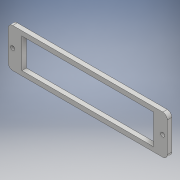
# Autodesk Inventor part: Frame
Saved by Autodesk Inventor 2017 (Build 210142000, 142)
## iProperties
Created: 2016-12-07
Part Number: Frame
Material: Generic
Document SubType Name: Modeling
Designer: willt
Density: 1 g/cm^3
Appearance: Default
Author: willt
Autodesk Inventor part; units mm, degrees
ref_plane "YZ Plane" through (0, 0, 0) normal (1, 0, 0) x (0, 1, 0)
ref_plane "XZ Plane" through (0, 0, 0) normal (0, 1, 0) x (-1, 0, 0)
ref_plane "XY Plane" through (0, 0, 0) normal (0, 0, 1) x (1, 0, 0)
sketch "Sketch2" plane through (0, 0, 0) normal (0, 1, 0) x (-1, 0, 0)
  line L0 (72.5, 16.5) -> (-72.5, 16.5)
  line L1 (-72.5, 16.5) -> (-72.5, -16.5)
  line L2 (-72.5, -16.5) -> (72.5, -16.5)
  line L3 (72.5, -16.5) -> (72.5, 16.5)
  line L4 (72.5, 16.5) -> (-72.5, -16.5) construction
  line L5 (-72.5, 16.5) -> (72.5, -16.5) construction
  line L6 (87.5, -21.5) -> (-87.5, -21.5)
  line L7 (-87.5, -21.5) -> (-87.5, 21.5)
  line L8 (-87.5, 21.5) -> (87.5, 21.5)
  line L9 (87.5, 21.5) -> (87.5, -21.5)
  line L10 (87.5, -21.5) -> (-87.5, 21.5) construction
  line L11 (-87.5, -21.5) -> (87.5, 21.5) construction
  line L12 (72.5, 0) -> (82.5, 0) construction
  circle A0 centre (82.5, 0) radius 2.25
  line L13 (0, -16.5) -> (0, 16.5)
  circle A1 centre (-82.5, 0) radius 2.25
  point P0 (0, 0)
  dimension "d12" = 145
  dimension "d13" = 33
  dimension "d14" = 175
  dimension "d15" = 43
  dimension "d16" = 10
  dimension "d17" = 4.5
  constraints: 28 end point, 7 midpoint, 4 parallel, 3 horizontal, 2 centre point, 2 perpendicular, 1 coincident, 1 symmetric about line, 1 other
  measures "d12" distance of L2.end L1.end
  measures "d13" distance of L1.end L0.end
  measures "d14" distance of L7.end L8.end
  measures "d15" distance of L6.end L7.end
  measures "d16" distance of L12.start L12.end
  measures "d17" diameter of A0
extrude "Extrusion2" add sketch "Sketch2" along normal blind 5
fillet "Fillet1" radius 5 1 edges at (87.5, 2.5, -21.5)
fillet "Fillet2" radius 5 3 edges at (87.5, 2.5, 21.5) (-87.5, 2.5, -21.5) (-87.5, 2.5, 21.5)
body "Solid2"
